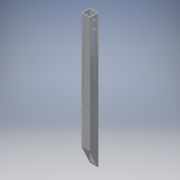
# Autodesk Inventor part: top
Saved by Autodesk Inventor 2016 (Build 200138000, 138)
## iProperties
Created: 2016-02-02
Part Number: top
Material: Aluminum 6061
Document SubType Name: Modeling
Designer: gus
Mass: 154.8 g
Surface Area: 727.399 cm^2
Volume: 57.3333 cm^3
Density: 2.7 g/cm^3
Appearance: Aluminum - Flat
Author: gus
Autodesk Inventor part; units mm, degrees
ref_plane "YZ Plane" through (0, 0, 0) normal (1, 0, 0) x (0, 1, 0)
ref_plane "XZ Plane" through (0, 0, 0) normal (0, 1, 0) x (-1, 0, 0)
ref_plane "XY Plane" through (0, 0, 0) normal (0, 0, 1) x (1, 0, 0)
sketch "Sketch1" plane through (0, 0, 0) normal (0, 1, 0) x (-1, 0, 0)
  line L0 (0, 0) -> (25.4, 0)
  line L1 (25.4, 0) -> (25.4, -25.4)
  line L2 (25.4, -25.4) -> (0, -25.4)
  line L3 (0, -25.4) -> (0, 0)
  line L4 (1.5875, -23.8125) -> (23.8125, -23.8125)
  line L5 (23.8125, -23.8125) -> (23.8125, -1.5875)
  line L6 (23.8125, -1.5875) -> (1.5875, -1.5875)
  line L7 (1.5875, -1.5875) -> (1.5875, -23.8125)
  dimension "d0" = 25.4
  dimension "d1" = 25.4
  dimension "d2" = 1.5875
  constraints: 16 end point, 4 parallel, 2 perpendicular, 1 horizontal, 3 other
  measures "d0" distance of L1.end L2.end
  measures "d1" distance of L0.end L1.end
  measures "d2" distance between parallel lines of L2 L4
extrude "Extrusion1" add sketch "Sketch1" along normal blind 406.4
sketch "Sketch2" plane through (0, 0, 0) normal (1, 0, 0) x (0, 0, -1)
  line L0 (25.4, 0) -> (25.4, 406.4) projected
  line L1 (25.4, 0) -> (0, 54.4705)
  line L2 (0, 0) -> (0, 406.4) projected
  line L3 (0, 54.4705) -> (0, 0)
  line L4 (0, 0) -> (25.4, 0)
  dimension "d5" = 25
  constraints: 6 end point, 1 collinear, 1 perpendicular, 1 point on line
  measures "d5" angle of L0 L1
extrude "Extrusion2" cut sketch "Sketch2" against normal blind 25.4
sketch "Sketch3" plane through (0, 406.4, 0) normal (1, 0, 0) x (0, 0, -1)
  circle A0 centre (12.7, -12.7) radius 3.3734
  line L0 (0, 0) -> (25.4, 0) projected
  line L1 (0, -351.9295) -> (0, 0) projected
  circle A1 centre (12.7, -38.1) radius 3.3734
  point P0 (0, -406.4)
  dimension "d8" = 6.7469
  dimension "d9" = 12.7
  dimension "d10" = 12.7
  dimension "d11" = 6.7469
  dimension "d12" = 12.7
  dimension "d13" = 38.1
  constraints: 2 centre point
  measures "d8" diameter of A0
  measures "d9" distance from line of L0 A0.centre
  measures "d10" distance from line of L1 A0.centre
  measures "d11" diameter of A1
  measures "d12" distance from line of L1 A1.centre
  measures "d13" distance from line of L0 A1.centre
extrude "Extrusion3" cut sketch "Sketch3" against normal blind 25.4
sketch "Sketch4" plane through (0, 406.4, 0) normal (1, 0, 0) x (0, 0, -1)
  circle A0 centre (12.7, -152.4) radius 3.3734
  line L0 (0, 0) -> (25.4, 0) projected
  circle A1 centre (12.7, -127) radius 3.3734
  circle A2 centre (12.7, -101.6) radius 3.3734
  line L1 (0, -351.9295) -> (0, 0) projected
  circle A3 centre (12.7, -247.65) radius 3.3734
  circle A4 centre (12.7, -222.25) radius 3.3734
  circle A5 centre (12.7, -273.05) radius 3.3734
  line L2 (12.7, -273.05) -> (12.7, -222.25) construction
  line L3 (25.4, -406.4) -> (25.4, 0) construction
  point P0 (0, -406.4)
  dimension "d16" = 6.7469
  dimension "d17" = 152.4
  dimension "d18" = 6.7469
  dimension "d19" = 25.4
  dimension "d20" = 6.7469
  dimension "d21" = 12.7
  dimension "d22" = 12.7
  dimension "d23" = 12.7
  dimension "d24" = 25.4
  dimension "d25" = 6.7469
  dimension "d26" = 25.4
  dimension "d27" = 25.4
  dimension "d28" = 12.7
  dimension "d30" = 273.05
  constraints: 6 centre point, 2 end point, 2 equal radius, 1 midpoint, 1 vertical
  measures "d16" diameter of A0
  measures "d17" distance from line of L0 A0.centre
  measures "d18" diameter of A1
  measures "d19" distance of A0.centre A1.centre
  measures "d20" diameter of A2
  measures "d21" distance from line of L1 A2.centre
  measures "d22" distance from line of L1 A1.centre
  measures "d23" distance from line of L1 A0.centre
  measures "d24" distance of A2.centre A1.centre
  measures "d25" diameter of A3
  measures "d26" distance of L2.end A3.centre
  measures "d27" distance of L2.start A3.centre
  measures "d28" distance between parallel lines of L3 L2
  measures "d30" distance from line of L0 L2.start
extrude "Extrusion4" cut sketch "Sketch4" against normal blind 25.4
body "Solid1"
